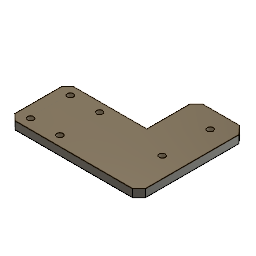
Y AXIX BELT (Autodesk Fusion 360 design; units mm, degrees)
Autodesk Fusion 360 part; units mm, degrees
sketch "Skizze1" plane through (0, 0, 0) normal (0, 1, 0) x (1, 0, 0)
  line L0 (0.076, -28.1203) -> (3.2508, -24.9466)
  line L1 (3.2508, -24.9466) -> (39.9722, -24.9466)
  line L2 (39.9722, -24.9466) -> (39.9722, -3.2655)
  line L3 (39.9722, -3.2655) -> (43.147, -0.076)
  line L4 (43.147, -0.076) -> (61.7964, -0.076)
  line L5 (61.7964, -0.076) -> (65.6865, -4.3091)
  line L6 (65.6865, -4.3091) -> (65.6863, -51.4541)
  line L7 (65.6863, -51.4541) -> (62.5115, -54.6291)
  line L8 (62.5115, -54.6291) -> (3.2509, -54.6291)
  line L9 (3.2509, -54.6291) -> (0.0761, -51.4721)
  line L10 (0.0761, -51.4721) -> (0.076, -28.1203)
  circle A0 centre (6.1496, -29.6153) radius 2.4004
  circle A1 centre (20.857, -29.6153) radius 2.4004
  circle A2 centre (6.1496, -49.6141) radius 2.4004
  circle A3 centre (20.857, -49.6141) radius 2.4004
  circle A4 centre (55.5723, -32.7901) radius 2.4004
  circle A5 centre (56.1634, -9.2632) radius 2.4004
  circle A6 centre (6.1496, -29.6153) radius 1.5
  circle A7 centre (6.1496, -49.6141) radius 1.5
  circle A8 centre (20.857, -29.6153) radius 1.5
  circle A9 centre (20.857, -49.6141) radius 1.5
  circle A10 centre (56.1634, -9.2632) radius 1.5
  circle A11 centre (55.5723, -32.7901) radius 1.5
  point P0 (8.55, -29.6153)
  point P1 (23.2574, -29.6153)
  point P2 (8.55, -49.6141)
  point P3 (23.2574, -49.6141)
  point P4 (57.9727, -32.7901)
  point P5 (58.5638, -9.2632)
  dimension "d1" = 3
  dimension "d2" = 3
  dimension "d3" = 3
  dimension "d4" = 3
  dimension "d5" = 3
  dimension "d6" = 3
  constraint concentric A0 A6
  constraint concentric A2 A7
  constraint concentric A1 A8
  constraint concentric A3 A9
  constraint concentric A5 A10
  constraint concentric A4 A11
  measures "d1" diameter of A6
  measures "d2" diameter of A7
  measures "d3" diameter of A8
  measures "d4" diameter of A9
  measures "d5" diameter of A10
  measures "d6" diameter of A11
extrude "Extrusion1" add sketch "Skizze1" along normal blind 4 contours L0 L1 L2 L3 L4 L5 L6 L7 L8 L9 L10 | A0 | A1 | A2 | A3 | A4 | A5
sketch "Skizze2" plane through (0, 4, 0) normal (0, 1, 0) x (-1, 0, 0)
  circle A0 centre (-55.5723, 32.7901) radius 1.5
  circle A1 centre (-20.857, 49.6141) radius 1.5
  circle A2 centre (-20.857, 29.6153) radius 1.5
  circle A3 centre (-6.1496, 49.6141) radius 1.5
  circle A4 centre (-56.1634, 9.2632) radius 1.5
  circle A5 centre (-6.1496, 29.6153) radius 1.5
  line L0 (-0.0761, 51.4721) -> (-3.2509, 54.6291)
  line L1 (-3.2509, 54.6291) -> (-62.5115, 54.6291)
  line L2 (-62.5115, 54.6291) -> (-65.6863, 51.4541)
  line L3 (-65.6863, 51.4541) -> (-65.6865, 4.3091)
  line L4 (-65.6865, 4.3091) -> (-61.7964, 0.076)
  line L5 (-61.7964, 0.076) -> (-43.147, 0.076)
  line L6 (-43.147, 0.076) -> (-39.9722, 3.2655)
  line L7 (-39.9722, 3.2655) -> (-39.9722, 24.9466)
  line L8 (-39.9722, 24.9466) -> (-3.2508, 24.9466)
  line L9 (-3.2508, 24.9466) -> (-0.076, 28.1203)
  line L10 (-0.076, 28.1203) -> (-0.0761, 51.4721)
sketch "Skizze3" plane through (0, 4, 0) normal (0, 1, 0) x (-1, 0, 0)
